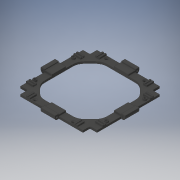
# Autodesk Inventor part: SoporteUNION_Rev.1
Saved by Autodesk Inventor 2019.1 (Build 231200000, 200)
## iProperties
Created: 2018-09-13
Part Number: SoporteUNION_Rev.1
Material: WindForm xt 2.0
Document SubType Name: Modeling
Designer: Elias
Density: 1.097 g/cm^3
Appearance: Genérico
Mass: 13.3352 g
Surface Area: 116.104 cm^2
Volume: 12.1561 cm^3
Author: Elias
Autodesk Inventor part; units mm, degrees
ref_plane "YZ Plane" through (0, 0, 0) normal (1, 0, 0) x (0, 1, 0)
ref_plane "XZ Plane" through (0, 0, 0) normal (0, 1, 0) x (-1, 0, 0)
sketch "Boceto1" plane through (0, 0, 0) normal (0, 1, 0) x (-1, 0, 0)
  line L0 (-40, 49) -> (40, 49)
  line L1 (49, 40) -> (49, -40)
  line L2 (40, -49) -> (-40, -49)
  line L3 (-49, -40) -> (-49, 40)
  line L4 (49, 49) -> (-49, -49) construction
  line L5 (40, 49) -> (40, 40)
  line L6 (40, 40) -> (49, 40)
  line L7 (40, -49) -> (40, -40)
  line L8 (40, -40) -> (49, -40)
  line L9 (-40, -49) -> (-40, -40)
  line L10 (-40, -40) -> (-49, -40)
  line L11 (-40, 49) -> (-40, 40)
  line L12 (-40, 40) -> (-49, 40)
  line L13 (24.3467, -40) -> (-24.3467, -40)
  line L14 (-40, -24.3467) -> (-40, 24.3467)
  line L15 (-24.3467, 40) -> (24.3467, 40)
  line L16 (40, 24.3467) -> (40, -24.3467)
  line L17 (40, -40) -> (-40, 40) construction
  line L18 (-40, -40) -> (40, 40) construction
  line L19 (-24.3467, -40) -> (-40, -24.3467)
  line L20 (40, 24.3467) -> (24.3467, 40)
  line L21 (24.3467, -40) -> (40, -24.3467)
  line L22 (-40, 24.3467) -> (-24.3467, 40)
  point P0 (0, 0)
  dimension "d2" = 9
  dimension "d3" = 9
  dimension "d4" = 9
  dimension "d5" = 9
  dimension "d6" = 9
  dimension "d7" = 9
  dimension "d8" = 9
  dimension "d9" = 9
  dimension "d10" = 49
  dimension "d11" = 49
  dimension "d15" = 80
  dimension "d16" = 80
  dimension "d17" = 91
  dimension "d18" = 45.5
  constraints: 46 end point, 6 parallel, 4 perpendicular, 3 midpoint, 2 horizontal
  measures "d2" distance of L1.start L5.end
  measures "d3" distance of L0.end L5.end
  measures "d4" distance of L1.end L7.end
  measures "d5" distance of L2.start L7.end
  measures "d6" distance of L3.start L9.end
  measures "d7" distance of L2.end L9.end
  measures "d8" distance of L3.end L11.end
  measures "d9" distance of L0.start L11.end
  measures "d10" distance from line of point (0, 0) L2
  measures "d11" distance from line of point (0, 0) L3
  measures "d15" distance of L18.start L17.end
  measures "d16" distance of L17.end L18.end
  measures "d17" distance between parallel lines of L20 L19
  measures "d18" distance from line of point (0, 0) L20
extrude "Extrusión2" add sketch "Boceto1" along normal blind 2.5
fillet "Empalme2" radius 1.5 4 edges at (40, 1.25, -40) (-40, 1.25, -40) (-40, 1.25, 40) (40, 1.25, 40)
fillet "Empalme2" radius 15 8 edges at (24.3467, 1.25, -40) (40, 1.25, -24.3467) (-24.3467, 1.25, -40) (-40, 1.25, -24.3467) (-40, 1.25, 24.3467) (24.3467, 1.25, 40) (40, 1.25, 24.3467) (-24.3467, 1.25, 40)
sketch "Boceto2" plane through (0, 2.5, 0) normal (0, 1, 0) x (1, 0, 0)
  circle A0 centre (24.7, -45.8) radius 1.25
  line L0 (49, -40) -> (49, 40) projected
  line L1 (-40, -49) -> (40, -49) projected
  line L2 (0, -49) -> (0, -40)
  circle A1 centre (-24.7, -45.8) radius 1.25
  line L3 (4.6367, 0) -> (-5.7922, 0)
  circle A2 centre (24.7, 45.8) radius 1.25
  circle A3 centre (-24.7, 45.8) radius 1.25
  point P0 (0, 0)
  dimension "d23" = 2.5
  dimension "d24" = 24.3
  dimension "d25" = 3.2
  constraints: 4 centre point, 4 end point, 3 symmetric about line, 1 horizontal, 1 midpoint, 1 vertical, 3 other
  measures "d23" diameter of A0
  measures "d24" distance from line of L0 A0.centre
  measures "d25" distance from line of L1 A0.centre
extrude "Extrusión3" cut sketch "Boceto2" against normal through all
sketch "Boceto3" plane through (0, 2.5, 0) normal (0, 1, 0) x (1, 0, 0)
  circle A0 centre (24.7, -45.8) radius 1.25 projected
  circle A1 centre (24.7, -45.8) radius 1.3
  circle A2 centre (24.7, -45.8) radius 2.25
  circle A3 centre (-24.7, -45.8) radius 1.25 projected
  circle A4 centre (-24.7, -45.8) radius 1.3
  circle A5 centre (-24.7, -45.8) radius 2.25
  line L0 (3.3315, 0) -> (-5.7248, 0)
  circle A6 centre (24.7, 45.8) radius 1.25
  circle A7 centre (24.7, 45.8) radius 1.3
  circle A8 centre (24.7, 45.8) radius 2.25
  circle A9 centre (-24.7, 45.8) radius 1.25
  circle A10 centre (-24.7, 45.8) radius 1.3
  circle A11 centre (-24.7, 45.8) radius 2.25
  point P0 (0, 0)
  dimension "d28" = 1
  dimension "d29" = 1
  constraints: 10 centre point, 4 coincident, 4 symmetric about line, 2 end point, 1 horizontal, 6 other
  measures "d28" radial gap between concentric circles of A0 A2
  measures "d29" radial gap between concentric circles of A3 A5
extrude "Extrusión4" add sketch "Boceto3" along normal blind 2 contours A1 | A2 | A4 | A5 | A7 | A8 | A10 | A11
sketch "Boceto4" plane through (18.1335, 2.5, 40) normal (0, 0, -1) x (-1, 0, 0)
  line L0 (36.267, -2.5) -> (0, -2.5) projected
  line L1 (9.1335, -2.5) -> (27.1335, -2.5)
  line L2 (27.1335, -2.5) -> (27.1335, 2)
  line L3 (27.1335, 2) -> (9.1335, 2)
  line L4 (9.1335, 2) -> (9.1335, -2.5)
  line L5 (58.1335, 0) -> (-21.8665, 0) projected
  line L6 (18.1335, 0) -> (18.1335, -2.5)
  dimension "d32" = 4.5
  dimension "d33" = 18
  dimension "d34" = 9
  constraints: 10 end point, 2 parallel, 1 horizontal, 1 midpoint, 1 perpendicular, 1 point on line, 1 vertical
  measures "d32" distance of L1.end L2.end
  measures "d33" distance of L2.end L3.end
  measures "d34" distance between parallel lines of L6 L2
extrude "Extrusión5" add sketch "Boceto4" against normal blind 13.9
sketch "Boceto5" plane through (-9, 4.5, 40) normal (0, 1, 0) x (1, 0, 0)
  line L0 (0, -13.9) -> (18, -13.9) projected
  line L1 (0, -9) -> (0, -13.9) projected
  line L2 (18, -13.9) -> (0, -13.9)
  line L3 (0, -13.9) -> (0, -9)
  line L4 (0, -9) -> (18, -9)
  line L5 (18, -9) -> (18, -13.9)
  point P0 (9, 40)
  constraints: 8 end point, 2 parallel, 1 horizontal, 1 perpendicular
extrude "Extrusión6" add sketch "Boceto5" along normal blind 1.1
sketch "Boceto6" plane through (-9, 2.5, 40) normal (-1, 0, 0) x (0, 0, 1)
  circle A0 centre (11.5, 0) radius 1.1
  line L0 (9, -2.5) -> (13.9, -2.5) projected
  line L1 (13.9, -2.5) -> (13.9, 3.1) projected
  point P0 (-40, -2.5)
  dimension "d39" = 2.2
  dimension "d40" = 2.5
  dimension "d41" = 2.4
  constraints: 1 centre point
  measures "d39" diameter of A0
  measures "d40" distance from line of L0 A0.centre
  measures "d41" distance from line of L1 A0.centre
extrude "Extrusión7" cut sketch "Boceto6" against normal through all
sketch "Boceto7" plane through (-9, 2.5, 40) normal (-1, 0, 0) x (0, 0, 1)
  line L0 (9, -2.5) -> (13.9, -2.5) projected
  line L1 (13.9, -2.5) -> (11.1, -2.5)
  line L2 (13.9, -2.5) -> (13.9, 0)
  line L3 (13.9, -2.5) -> (13.9, 3.1) projected
  ellipse E0 centre (11.1, 0) end of major axis (11.1, -2.5) minor radius 2.8 (11.1, -2.5) -> (13.9, 0) ccw
  point P0 (-40, -2.5)
  dimension "d44" = 2.8
  dimension "d45" = 2.5
  constraints: 4 end point, 2 point on line, 4 other
  measures "d44" distance of L0.end L1.end
  measures "d45" distance of L0.end L2.end
extrude "Extrusión8" cut sketch "Boceto7" against normal through all
sketch "Boceto8" plane through (-40, 0, 49) normal (0, 0, 1) x (1, 0, 0)
  line L0 (0, 0) -> (0, 2.5) projected
  line L1 (12, 2.5) -> (12, 4.5)
  line L2 (12, 4.5) -> (7, 4.5)
  line L3 (7, 4.5) -> (7, 2.5)
  line L4 (7, 2.5) -> (8.5, 2.5)
  line L5 (10.5, 2.5) -> (12, 2.5)
  line L6 (31, 5.6) -> (49, 5.6) projected
  line L7 (40, 5.6) -> (40, 0)
  line L8 (68, 2.5) -> (68, 4.5)
  line L9 (68, 4.5) -> (73, 4.5)
  line L10 (73, 4.5) -> (73, 2.5)
  line L11 (73, 2.5) -> (71.5, 2.5)
  line L12 (69.5, 2.5) -> (68, 2.5)
  line L13 (31, 2.5) -> (31, 0) projected
  line L14 (0, 2.5) -> (31, 2.5) projected
  line L15 (8.5, 2.5) -> (10.5, 2.5)
  line L16 (80, 2.5) -> (0, 2.5) projected
  line L17 (69.5, 2.5) -> (71.5, 2.5)
  dimension "d53" = 2
  dimension "d54" = 5
  dimension "d86" = 0
  dimension "d87" = 0
  dimension "d92" = 7
  constraints: 26 end point, 6 symmetric about line, 3 parallel, 2 horizontal, 2 perpendicular, 1 midpoint, 1 vertical, 1 other
  measures "d53" distance of L2.end L3.end
  measures "d54" distance of L1.end L2.end
  measures "d86" distance between parallel lines of L14 L5
  measures "d87" distance between parallel lines of L14 L4
  measures "d92" distance between parallel lines of L0 L3
extrude "Extrusión9" add sketch "Boceto8" against normal blind 9
pattern_circular "Patrón circular1" count 4 over 360 about axis through (0, -10, 0) along (0, 1, 0) of "Extrusión5", "Extrusión6", "Extrusión7", "Extrusión8", "Extrusión9"
pattern_circular "Patrón circular2" count 2 over 90 about axis through (0, -10, 0) along (0, 1, 0) of "Extrusión4"
sketch "Boceto10" plane through (49, 4.5, -28) normal (0, 1, 0) x (1, 0, 0)
  line L0 (-19.25, -81.1589) -> (-17.75, -81.1589)
  line L1 (-17.75, -81.1589) -> (-17.75, -63.1589)
  line L2 (-19.25, -63.1589) -> (-19.25, -81.1589)
  line L3 (-19.25, -81.1589) -> (-17.75, -63.1589) construction
  line L4 (-17.75, -81.1589) -> (-19.25, -63.1589) construction
  line L5 (-19.25, -63.1589) -> (-17.75, -63.1589)
  line L6 (-16, -77) -> (-16, -68) projected
  point P0 (-49, -28)
  point P1 (-18.5, -72.1589)
  dimension "d157" = 1.5
  dimension "d159" = 2.5
  constraints: 12 end point, 1 horizontal, 1 midpoint, 1 parallel, 1 perpendicular
  measures "d157" distance of L0.start L0.end
  measures "d159" distance from line of point (-18.5, -72.159) L6
extrude "Extrusión11" cut sketch "Boceto10" against normal blind 1
sketch "Boceto11" plane through (-49, 4.5, -9) normal (1, 0, 0) x (0, 0, -1)
  line L0 (0, 0) -> (-18, 0) projected
  line L1 (0, 0) -> (0, 1.1) projected
  line L2 (-18, 1.1) -> (0, 1.1) projected
  line L3 (-18, 0) -> (-18, 1.1) projected
  point P0 (-9, -4.5)
extrude "Extrusión12" cut sketch "Boceto11" against normal blind 0.2
pattern_circular "Patrón circular3" count 4 over 360 about axis through (0, -10, 0) along (0, 1, 0) of "Extrusión12"
sketch "Boceto12" plane through (-45.8, 2.5, 24.7) normal (0, 1, 0) x (1, 0, 0)
  circle A0 centre (0, 0) radius 1.25 projected
  circle A1 centre (0, 49.4) radius 1.25 projected
  circle A2 centre (91.6, 49.4) radius 1.25 projected
  circle A3 centre (91.6, 0) radius 1.25 projected
  point P0 (45.8, 24.7)
extrude "Extrusión13" cut sketch "Boceto12" against normal blind 10
ref_plane "Plano de trabajo2" through (-33, 4.5, 49) normal (0, 1, 0) x (1, 0, 0)
sketch "Boceto13" plane through (-33, 4.5, 49) normal (0, 1, 0) x (1, 0, 0)
  line L0 (1.75, 27) -> (3.25, 27)
  line L1 (3.25, 27) -> (3.25, 0)
  line L2 (3.25, 0) -> (1.75, 0)
  line L3 (1.75, 0) -> (1.75, 27)
  line L4 (1.75, 27) -> (3.25, 0) construction
  line L5 (3.25, 27) -> (1.75, 0) construction
  line L6 (5, 0) -> (5, 9) projected
  point P0 (33, 49)
  point P1 (2.5, 13.5)
  dimension "d111" = 1.5
  dimension "d156" = 2.5
  constraints: 12 end point, 2 parallel, 1 horizontal, 1 midpoint, 1 perpendicular
  measures "d111" distance of L1.end L2.end
  measures "d156" distance from line of point (2.5, 13.5) L6
extrude "Extrusión14" cut sketch "Boceto13" against normal blind 1
pattern_circular "Patrón circular5" count 4 over 360 about axis through (0, -10, 0) along (0, 1, 0) of "Extrusión14"
sketch "Boceto14" plane through (24.7, 4.5, 45.8) normal (0, 1, 0) x (1, 0, 0)
  circle A0 centre (-49.4, 0) radius 1.25 projected
  circle A1 centre (-49.4, 0) radius 2.25 projected
  circle A2 centre (0, 0) radius 2.25 projected
  circle A3 centre (-49.4, 91.6) radius 2.25 projected
  circle A4 centre (0, 91.6) radius 2.25 projected
  point P0 (-24.7, 45.8)
extrude "Extrusión15" cut sketch "Boceto14" against normal up to surface (2 mm away) contours A0 | A1 | A2 | A3 | A4
sketch "Boceto15" plane through (0, 2.5, 0) normal (0, 1, 0) x (1, 0, 0)
  circle A0 centre (-24.7, -45.8) radius 1.25 projected
  point P0 (0, 0)
  constraints: 1 coincident
hole "Agujero1" at (-24.7, 2.5, 45.8) direction (0, -1, 0) diameter 2.6 end through all countersink diameter 4.7 countersink angle 90
sketch "Boceto16" plane through (0, 2.5, 0) normal (0, 1, 0) x (1, 0, 0)
  circle A0 centre (24.7, -45.8) radius 1.25 projected
  point P0 (0, 0)
  constraints: 1 coincident
hole "Agujero2" at (24.7, 2.5, 45.8) direction (0, -1, 0) diameter 2.6 end through all countersink diameter 4.7 countersink angle 90
sketch "Boceto17" plane through (0, 2.5, 0) normal (0, 1, 0) x (1, 0, 0)
  circle A0 centre (24.7, 45.8) radius 1.25 projected
  point P0 (0, 0)
  constraints: 1 coincident
hole "Agujero3" at (24.7, 2.5, -45.8) direction (0, -1, 0) diameter 2.6 end through all countersink diameter 4.7 countersink angle 90
sketch "Boceto18" plane through (0, 2.5, 0) normal (0, 1, 0) x (1, 0, 0)
  circle A0 centre (-24.7, 45.8) radius 1.25 projected
  point P0 (0, 0)
  constraints: 1 coincident
hole "Agujero4" at (-24.7, 2.5, -45.8) direction (0, -1, 0) diameter 2.6 end through all countersink diameter 4.7 countersink angle 90
pattern_circular "Patrón circular6" count 4 over 360 about axis through (0, -10, 0) along (0, 1, 0) of "Extrusión11"
